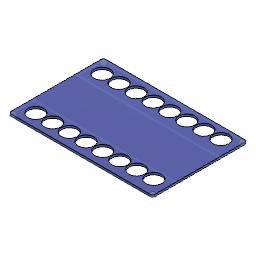
top1 (Autodesk Fusion 360 design; units mm, degrees)
part number: 2025-09-26-14-14-50-476
Autodesk Fusion 360 part; units mm, degrees
sketch "Sketch1" plane through (0, 0, 0) normal (0, 0, 1) x (1, 0, 0)
  line L0 (5, 0) -> (306, 0)
  line L1 (311, 5) -> (311, 200)
  line L2 (306, 205) -> (5, 205)
  line L3 (0, 200) -> (0, 5)
  circle A0 centre (30, 29) radius 17
  circle A1 centre (65.8571, 29.3) radius 17
  circle A2 centre (101.7143, 29.6) radius 17
  circle A3 centre (28, 174) radius 17
  circle A4 centre (99.7143, 176) radius 17
  circle A5 centre (63.8571, 175) radius 17
  circle A6 centre (137.5714, 29.9) radius 17
  circle A7 centre (135.5714, 177) radius 17
  circle A8 centre (173.4286, 30.1) radius 17
  circle A9 centre (209.2857, 31) radius 17
  circle A10 centre (245.1429, 32) radius 17
  circle A11 centre (281, 33) radius 17
  circle A12 centre (171.4286, 177) radius 17
  circle A13 centre (207.2857, 178) radius 17
  circle A14 centre (243.1429, 179) radius 17
  circle A15 centre (279, 180) radius 17
  arc A16 (311, 200) -> (306, 205) centre (306, 200) ccw
  arc A17 (5, 205) -> (0, 200) centre (5, 200) ccw
  arc A18 (306, 0) -> (311, 5) centre (306, 5) ccw
  arc A19 (0, 5) -> (5, 0) centre (5, 5) ccw
  dimension "d1" = 311
  dimension "d2" = 205
  dimension "d4" = 34
  dimension "d6" = 29
  dimension "d8" = 34
  dimension "d9" = 34
  dimension "d10" = 34
  dimension "d11" = 34
  dimension "d13" = 34
  dimension "d14" = 34
  dimension "d15" = 34
  dimension "d16" = 34
  dimension "d17" = 34
  dimension "d18" = 34
  dimension "d19" = 34
  dimension "d28" = 29.3
  dimension "d29" = 29.6
  dimension "d30" = 29.9
  dimension "d31" = 30.1
  dimension "d32" = 31
  dimension "d33" = 32
  dimension "d34" = 33
  dimension "d35" = 34
  dimension "d36" = 34
  dimension "d37" = 34
  dimension "d38" = 34
  dimension "d48" = 31
  dimension "d49" = 30
  dimension "d50" = 29
  dimension "d51" = 28
  dimension "d52" = 28
  dimension "d53" = 27
  dimension "d55" = 30
  dimension "d56" = 35.8571
  dimension "d57" = 35.8571
  dimension "d58" = 35.8571
  dimension "d59" = 35.8571
  dimension "d60" = 35.8571
  dimension "d61" = 35.8571
  dimension "d62" = 35.8571
  dimension "d63" = 30
  dimension "d64" = 28
  dimension "d66" = 35.8571
  dimension "d67" = 35.8571
  dimension "d68" = 35.8571
  dimension "d69" = 35.8571
  dimension "d70" = 35.8571
  dimension "d71" = 35.8571
  dimension "d72" = 32
  dimension "d73" = 26
  dimension "d74" = 25
  dimension "d75" = 35.8571
  dimension "d76" = 5
  dimension "d77" = 5
  dimension "d78" = 5
  dimension "d79" = 5
  constraint horizontal L0
  constraint vertical L1
  constraint horizontal L2
  constraint vertical L3
  constraint tangent L1 A16
  constraint tangent L2 A16
  constraint tangent L2 A17
  constraint tangent L3 A17
  constraint tangent L0 A18
  constraint tangent L1 A18
  constraint tangent L0 A19
  constraint tangent L3 A19
  measures "d1" distance of L1 L3
  measures "d2" distance of L0 L2
  measures "d4" diameter of A0
  measures "d6" distance of L0 A0.centre
  measures "d8" diameter of A1
  measures "d9" diameter of A2
  measures "d10" diameter of A3
  measures "d11" diameter of A4
  measures "d13" diameter of A5
  measures "d14" diameter of A6
  measures "d15" diameter of A7
  measures "d16" diameter of A8
  measures "d17" diameter of A9
  measures "d18" diameter of A10
  measures "d19" diameter of A11
  measures "d28" distance of L0 A1.centre
  measures "d29" distance of L0 A2.centre
  measures "d30" distance of L0 A6.centre
  measures "d31" distance of L0 A8.centre
  measures "d32" distance of L0 A9.centre
  measures "d33" distance of L0 A10.centre
  measures "d34" distance of L0 A11.centre
  measures "d35" diameter of A12
  measures "d36" diameter of A13
  measures "d37" diameter of A14
  measures "d38" diameter of A15
  measures "d48" distance of L2 A3.centre
  measures "d49" distance of L2 A5.centre
  measures "d50" distance of L2 A4.centre
  measures "d51" distance of L2 A7.centre
  measures "d52" distance of L2 A12.centre
  measures "d53" distance of L2 A13.centre
  measures "d55" distance of L3 A0.centre
  measures "d56" horizontal distance of A0.centre A1.centre
  measures "d57" horizontal distance of A1.centre A2.centre
  measures "d58" horizontal distance of A2.centre A6.centre
  measures "d59" horizontal distance of A6.centre A8.centre
  measures "d60" horizontal distance of A8.centre A9.centre
  measures "d61" horizontal distance of A9.centre A10.centre
  measures "d62" horizontal distance of A10.centre A11.centre
  measures "d63" distance of L1 A11.centre
  measures "d64" distance of L3 A3.centre
  measures "d66" horizontal distance of A4.centre A5.centre
  measures "d67" horizontal distance of A4.centre A7.centre
  measures "d68" horizontal distance of A7.centre A12.centre
  measures "d69" horizontal distance of A12.centre A13.centre
  measures "d70" horizontal distance of A13.centre A14.centre
  measures "d71" horizontal distance of A14.centre A15.centre
  measures "d72" distance of L1 A15.centre
  measures "d73" distance of L2 A14.centre
  measures "d74" distance of L2 A15.centre
  measures "d75" horizontal distance of A3.centre A5.centre
  measures "d76" radius of A16
  measures "d77" radius of A17
  measures "d78" radius of A18
  measures "d79" radius of A19
sketch "Sketch2" plane through (0, 0, 0) normal (0, 0, 1) x (1, 0, 0)
extrude "Extrude1" add sketch "Sketch1" along normal blind 3.5
extrude "Extrude2" add 1 faces at (123.0248, 122.1087, 3.5) along direction (0, 0, 1) blind 1
sketch "Sketch3" plane through (0, 0, 0) normal (0, 0, 1) x (1, 0, 0)
  line L0 (5, 0) -> (306.1184, 0)
  line L1 (311.1184, 5) -> (311.1184, 55.2879)
  line L2 (311.1184, 55.2879) -> (0, 55.2879)
  line L3 (0, 55.2879) -> (0, 5)
  line L4 (310, 148.1101) -> (0, 148.1101)
  line L5 (0, 148.1101) -> (0, 199.7882)
  line L6 (5, 204.7882) -> (305, 204.7882)
  line L7 (310, 199.7882) -> (310, 148.1101)
  arc A0 (5, 204.7882) -> (0, 199.7882) centre (5, 199.7882) ccw
  arc A1 (310, 199.7882) -> (305, 204.7882) centre (305, 199.7882) ccw
  arc A2 (0, 5) -> (5, 0) centre (5, 5) ccw
  arc A3 (306.1184, 0) -> (311.1184, 5) centre (306.1184, 5) ccw
  dimension "d84" = 5
  dimension "d85" = 5
  dimension "d86" = 5
  dimension "d87" = 5
  constraint horizontal L0
  constraint vertical L1
  constraint horizontal L2
  constraint vertical L3
  constraint horizontal L4
  constraint vertical L5
  constraint horizontal L6
  constraint vertical L7
  constraint tangent L5 A0
  constraint tangent L6 A0
  constraint tangent L6 A1
  constraint tangent L7 A1
  constraint tangent L0 A2
  constraint tangent L3 A2
  constraint tangent L0 A3
  constraint tangent L1 A3
  measures "d84" radius of A0
  measures "d85" radius of A1
  measures "d86" radius of A2
  measures "d87" radius of A3
sketch "Sketch4" plane through (0, 0, 0) normal (0, 0, 1) x (1, 0, 0)
